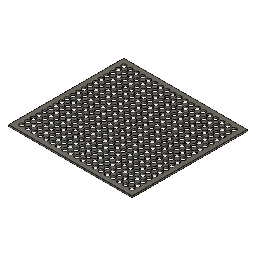
Top (Autodesk Fusion 360 design; units mm, degrees)
Autodesk Fusion 360 part; units mm, degrees
sketch "Sketch1" plane through (0, 0, 0) normal (0, 0, 1) x (1, 0, 0)
  circle A0 centre (11.85, 11) radius 9
  circle A1 centre (35.55, 11) radius 9
  circle A2 centre (59.25, 11) radius 9
  circle A3 centre (82.95, 11) radius 9
  circle A4 centre (106.65, 11) radius 9
  circle A5 centre (130.35, 11) radius 9
  circle A6 centre (154.05, 11) radius 9
  circle A7 centre (177.75, 11) radius 9
  circle A8 centre (201.45, 11) radius 9
  circle A9 centre (225.15, 11) radius 9
  circle A10 centre (248.85, 11) radius 9
  circle A11 centre (272.55, 11) radius 9
  circle A12 centre (296.25, 11) radius 9
  circle A13 centre (319.95, 11) radius 9
  circle A14 centre (343.65, 11) radius 9
  circle A15 centre (367.35, 11) radius 9
  circle A16 centre (391.05, 11) radius 9
  circle A17 centre (414.75, 11) radius 9
  circle A18 centre (438.45, 11) radius 9
  circle A19 centre (11.85, 33) radius 9
  circle A20 centre (35.55, 33) radius 9
  circle A21 centre (59.25, 33) radius 9
  circle A22 centre (82.95, 33) radius 9
  circle A23 centre (106.65, 33) radius 9
  circle A24 centre (130.35, 33) radius 9
  circle A25 centre (154.05, 33) radius 9
  circle A26 centre (177.75, 33) radius 9
  circle A27 centre (201.45, 33) radius 9
  circle A28 centre (225.15, 33) radius 9
  circle A29 centre (248.85, 33) radius 9
  circle A30 centre (272.55, 33) radius 9
  circle A31 centre (296.25, 33) radius 9
  circle A32 centre (319.95, 33) radius 9
  circle A33 centre (343.65, 33) radius 9
  circle A34 centre (367.35, 33) radius 9
  circle A35 centre (391.05, 33) radius 9
  circle A36 centre (414.75, 33) radius 9
  circle A37 centre (438.45, 33) radius 9
  circle A38 centre (11.85, 55) radius 9
  circle A39 centre (35.55, 55) radius 9
  circle A40 centre (59.25, 55) radius 9
  circle A41 centre (82.95, 55) radius 9
  circle A42 centre (106.65, 55) radius 9
  circle A43 centre (130.35, 55) radius 9
  circle A44 centre (154.05, 55) radius 9
  circle A45 centre (177.75, 55) radius 9
  circle A46 centre (201.45, 55) radius 9
  circle A47 centre (225.15, 55) radius 9
  circle A48 centre (248.85, 55) radius 9
  circle A49 centre (272.55, 55) radius 9
  circle A50 centre (296.25, 55) radius 9
  circle A51 centre (319.95, 55) radius 9
  circle A52 centre (343.65, 55) radius 9
  circle A53 centre (367.35, 55) radius 9
  circle A54 centre (391.05, 55) radius 9
  circle A55 centre (414.75, 55) radius 9
  circle A56 centre (438.45, 55) radius 9
  circle A57 centre (11.85, 77) radius 9
  circle A58 centre (35.55, 77) radius 9
  circle A59 centre (59.25, 77) radius 9
  circle A60 centre (82.95, 77) radius 9
  circle A61 centre (106.65, 77) radius 9
  circle A62 centre (130.35, 77) radius 9
  circle A63 centre (154.05, 77) radius 9
  circle A64 centre (177.75, 77) radius 9
  circle A65 centre (201.45, 77) radius 9
  circle A66 centre (225.15, 77) radius 9
  circle A67 centre (248.85, 77) radius 9
  circle A68 centre (272.55, 77) radius 9
  circle A69 centre (296.25, 77) radius 9
  circle A70 centre (319.95, 77) radius 9
  circle A71 centre (343.65, 77) radius 9
  circle A72 centre (367.35, 77) radius 9
  circle A73 centre (391.05, 77) radius 9
  circle A74 centre (414.75, 77) radius 9
  circle A75 centre (438.45, 77) radius 9
  circle A76 centre (11.85, 99) radius 9
  circle A77 centre (35.55, 99) radius 9
  circle A78 centre (59.25, 99) radius 9
  circle A79 centre (82.95, 99) radius 9
  circle A80 centre (106.65, 99) radius 9
  circle A81 centre (130.35, 99) radius 9
  circle A82 centre (154.05, 99) radius 9
  circle A83 centre (177.75, 99) radius 9
  circle A84 centre (201.45, 99) radius 9
  circle A85 centre (225.15, 99) radius 9
  circle A86 centre (248.85, 99) radius 9
  circle A87 centre (272.55, 99) radius 9
  circle A88 centre (296.25, 99) radius 9
  circle A89 centre (319.95, 99) radius 9
  circle A90 centre (343.65, 99) radius 9
  circle A91 centre (367.35, 99) radius 9
  circle A92 centre (391.05, 99) radius 9
  circle A93 centre (414.75, 99) radius 9
  circle A94 centre (438.45, 99) radius 9
  circle A95 centre (11.85, 121) radius 9
  circle A96 centre (35.55, 121) radius 9
  circle A97 centre (59.25, 121) radius 9
  circle A98 centre (82.95, 121) radius 9
  circle A99 centre (106.65, 121) radius 9
  circle A100 centre (130.35, 121) radius 9
  circle A101 centre (154.05, 121) radius 9
  circle A102 centre (177.75, 121) radius 9
  circle A103 centre (201.45, 121) radius 9
  circle A104 centre (225.15, 121) radius 9
  circle A105 centre (248.85, 121) radius 9
  circle A106 centre (272.55, 121) radius 9
  circle A107 centre (296.25, 121) radius 9
  circle A108 centre (319.95, 121) radius 9
  circle A109 centre (343.65, 121) radius 9
  circle A110 centre (367.35, 121) radius 9
  circle A111 centre (391.05, 121) radius 9
  circle A112 centre (414.75, 121) radius 9
  circle A113 centre (438.45, 121) radius 9
  circle A114 centre (11.85, 143) radius 9
  circle A115 centre (35.55, 143) radius 9
  circle A116 centre (59.25, 143) radius 9
  circle A117 centre (82.95, 143) radius 9
  circle A118 centre (106.65, 143) radius 9
  circle A119 centre (130.35, 143) radius 9
  circle A120 centre (154.05, 143) radius 9
  circle A121 centre (177.75, 143) radius 9
  circle A122 centre (201.45, 143) radius 9
  circle A123 centre (225.15, 143) radius 9
  circle A124 centre (248.85, 143) radius 9
  circle A125 centre (272.55, 143) radius 9
  circle A126 centre (296.25, 143) radius 9
  circle A127 centre (319.95, 143) radius 9
  circle A128 centre (343.65, 143) radius 9
  circle A129 centre (367.35, 143) radius 9
  circle A130 centre (391.05, 143) radius 9
  circle A131 centre (414.75, 143) radius 9
  circle A132 centre (438.45, 143) radius 9
  circle A133 centre (11.85, 165) radius 9
  circle A134 centre (35.55, 165) radius 9
  circle A135 centre (59.25, 165) radius 9
  circle A136 centre (82.95, 165) radius 9
  circle A137 centre (106.65, 165) radius 9
  circle A138 centre (130.35, 165) radius 9
  circle A139 centre (154.05, 165) radius 9
  circle A140 centre (177.75, 165) radius 9
  circle A141 centre (201.45, 165) radius 9
  circle A142 centre (225.15, 165) radius 9
  circle A143 centre (248.85, 165) radius 9
  circle A144 centre (272.55, 165) radius 9
  circle A145 centre (296.25, 165) radius 9
  circle A146 centre (319.95, 165) radius 9
  circle A147 centre (343.65, 165) radius 9
  circle A148 centre (367.35, 165) radius 9
  circle A149 centre (391.05, 165) radius 9
  circle A150 centre (414.75, 165) radius 9
  circle A151 centre (438.45, 165) radius 9
  circle A152 centre (11.85, 187) radius 9
  circle A153 centre (35.55, 187) radius 9
  circle A154 centre (59.25, 187) radius 9
  circle A155 centre (82.95, 187) radius 9
  circle A156 centre (106.65, 187) radius 9
  circle A157 centre (130.35, 187) radius 9
  circle A158 centre (154.05, 187) radius 9
  circle A159 centre (177.75, 187) radius 9
  circle A160 centre (201.45, 187) radius 9
  circle A161 centre (225.15, 187) radius 9
  circle A162 centre (248.85, 187) radius 9
  circle A163 centre (272.55, 187) radius 9
  circle A164 centre (296.25, 187) radius 9
  circle A165 centre (319.95, 187) radius 9
  circle A166 centre (343.65, 187) radius 9
  circle A167 centre (367.35, 187) radius 9
  circle A168 centre (391.05, 187) radius 9
  circle A169 centre (414.75, 187) radius 9
  circle A170 centre (438.45, 187) radius 9
  circle A171 centre (11.85, 209) radius 9
  circle A172 centre (35.55, 209) radius 9
  circle A173 centre (59.25, 209) radius 9
  circle A174 centre (82.95, 209) radius 9
  circle A175 centre (106.65, 209) radius 9
  circle A176 centre (130.35, 209) radius 9
  circle A177 centre (154.05, 209) radius 9
  circle A178 centre (177.75, 209) radius 9
  circle A179 centre (201.45, 209) radius 9
  circle A180 centre (225.15, 209) radius 9
  circle A181 centre (248.85, 209) radius 9
  circle A182 centre (272.55, 209) radius 9
  circle A183 centre (296.25, 209) radius 9
  circle A184 centre (319.95, 209) radius 9
  circle A185 centre (343.65, 209) radius 9
  circle A186 centre (367.35, 209) radius 9
  circle A187 centre (391.05, 209) radius 9
  circle A188 centre (414.75, 209) radius 9
  circle A189 centre (438.45, 209) radius 9
  circle A190 centre (11.85, 231) radius 9
  circle A191 centre (35.55, 231) radius 9
  circle A192 centre (59.25, 231) radius 9
  circle A193 centre (82.95, 231) radius 9
  circle A194 centre (106.65, 231) radius 9
  circle A195 centre (130.35, 231) radius 9
  circle A196 centre (154.05, 231) radius 9
  circle A197 centre (177.75, 231) radius 9
  circle A198 centre (201.45, 231) radius 9
  circle A199 centre (225.15, 231) radius 9
  circle A200 centre (248.85, 231) radius 9
  circle A201 centre (272.55, 231) radius 9
  circle A202 centre (296.25, 231) radius 9
  circle A203 centre (319.95, 231) radius 9
  circle A204 centre (343.65, 231) radius 9
  circle A205 centre (367.35, 231) radius 9
  circle A206 centre (391.05, 231) radius 9
  circle A207 centre (414.75, 231) radius 9
  circle A208 centre (438.45, 231) radius 9
  circle A209 centre (11.85, 253) radius 9
  circle A210 centre (35.55, 253) radius 9
  circle A211 centre (59.25, 253) radius 9
  circle A212 centre (82.95, 253) radius 9
  circle A213 centre (106.65, 253) radius 9
  circle A214 centre (130.35, 253) radius 9
  circle A215 centre (154.05, 253) radius 9
  circle A216 centre (177.75, 253) radius 9
  circle A217 centre (201.45, 253) radius 9
  circle A218 centre (225.15, 253) radius 9
  circle A219 centre (248.85, 253) radius 9
  circle A220 centre (272.55, 253) radius 9
  circle A221 centre (296.25, 253) radius 9
  circle A222 centre (319.95, 253) radius 9
  circle A223 centre (343.65, 253) radius 9
  circle A224 centre (367.35, 253) radius 9
  circle A225 centre (391.05, 253) radius 9
  circle A226 centre (414.75, 253) radius 9
  circle A227 centre (438.45, 253) radius 9
  circle A228 centre (11.85, 275) radius 9
  circle A229 centre (35.55, 275) radius 9
  circle A230 centre (59.25, 275) radius 9
  circle A231 centre (82.95, 275) radius 9
  circle A232 centre (106.65, 275) radius 9
  circle A233 centre (130.35, 275) radius 9
  circle A234 centre (154.05, 275) radius 9
  circle A235 centre (177.75, 275) radius 9
  circle A236 centre (201.45, 275) radius 9
  circle A237 centre (225.15, 275) radius 9
  circle A238 centre (248.85, 275) radius 9
  circle A239 centre (272.55, 275) radius 9
  circle A240 centre (296.25, 275) radius 9
  circle A241 centre (319.95, 275) radius 9
  circle A242 centre (343.65, 275) radius 9
  circle A243 centre (367.35, 275) radius 9
  circle A244 centre (391.05, 275) radius 9
  circle A245 centre (414.75, 275) radius 9
  circle A246 centre (438.45, 275) radius 9
  circle A247 centre (11.85, 297) radius 9
  circle A248 centre (35.55, 297) radius 9
  circle A249 centre (59.25, 297) radius 9
  circle A250 centre (82.95, 297) radius 9
  circle A251 centre (106.65, 297) radius 9
  circle A252 centre (130.35, 297) radius 9
  circle A253 centre (154.05, 297) radius 9
  circle A254 centre (177.75, 297) radius 9
  circle A255 centre (201.45, 297) radius 9
  circle A256 centre (225.15, 297) radius 9
  circle A257 centre (248.85, 297) radius 9
  circle A258 centre (272.55, 297) radius 9
  circle A259 centre (296.25, 297) radius 9
  circle A260 centre (319.95, 297) radius 9
  circle A261 centre (343.65, 297) radius 9
  circle A262 centre (367.35, 297) radius 9
  circle A263 centre (391.05, 297) radius 9
  circle A264 centre (414.75, 297) radius 9
  circle A265 centre (438.45, 297) radius 9
  circle A266 centre (11.85, 319) radius 9
  circle A267 centre (35.55, 319) radius 9
  circle A268 centre (59.25, 319) radius 9
  circle A269 centre (82.95, 319) radius 9
  circle A270 centre (106.65, 319) radius 9
  circle A271 centre (130.35, 319) radius 9
  circle A272 centre (154.05, 319) radius 9
  circle A273 centre (177.75, 319) radius 9
  circle A274 centre (201.45, 319) radius 9
  circle A275 centre (225.15, 319) radius 9
  circle A276 centre (248.85, 319) radius 9
  circle A277 centre (272.55, 319) radius 9
  circle A278 centre (296.25, 319) radius 9
  circle A279 centre (319.95, 319) radius 9
  circle A280 centre (343.65, 319) radius 9
  circle A281 centre (367.35, 319) radius 9
  circle A282 centre (391.05, 319) radius 9
  circle A283 centre (414.75, 319) radius 9
  circle A284 centre (438.45, 319) radius 9
  circle A285 centre (11.85, 341) radius 9
  circle A286 centre (35.55, 341) radius 9
  circle A287 centre (59.25, 341) radius 9
  circle A288 centre (82.95, 341) radius 9
  circle A289 centre (106.65, 341) radius 9
  circle A290 centre (130.35, 341) radius 9
  circle A291 centre (154.05, 341) radius 9
  circle A292 centre (177.75, 341) radius 9
  circle A293 centre (201.45, 341) radius 9
  circle A294 centre (225.15, 341) radius 9
  circle A295 centre (248.85, 341) radius 9
  circle A296 centre (272.55, 341) radius 9
  circle A297 centre (296.25, 341) radius 9
  circle A298 centre (319.95, 341) radius 9
  circle A299 centre (343.65, 341) radius 9
  circle A300 centre (367.35, 341) radius 9
  circle A301 centre (391.05, 341) radius 9
  circle A302 centre (414.75, 341) radius 9
  circle A303 centre (438.45, 341) radius 9
  circle A304 centre (11.85, 363) radius 9
  circle A305 centre (35.55, 363) radius 9
  circle A306 centre (59.25, 363) radius 9
  circle A307 centre (82.95, 363) radius 9
  circle A308 centre (106.65, 363) radius 9
  circle A309 centre (130.35, 363) radius 9
  circle A310 centre (154.05, 363) radius 9
  circle A311 centre (177.75, 363) radius 9
  circle A312 centre (201.45, 363) radius 9
  circle A313 centre (225.15, 363) radius 9
  circle A314 centre (248.85, 363) radius 9
  circle A315 centre (272.55, 363) radius 9
  circle A316 centre (296.25, 363) radius 9
  circle A317 centre (319.95, 363) radius 9
  circle A318 centre (343.65, 363) radius 9
  circle A319 centre (367.35, 363) radius 9
  circle A320 centre (391.05, 363) radius 9
  circle A321 centre (414.75, 363) radius 9
  circle A322 centre (438.45, 363) radius 9
  circle A323 centre (11.85, 385) radius 9
  circle A324 centre (35.55, 385) radius 9
  circle A325 centre (59.25, 385) radius 9
  circle A326 centre (82.95, 385) radius 9
  circle A327 centre (106.65, 385) radius 9
  circle A328 centre (130.35, 385) radius 9
  circle A329 centre (154.05, 385) radius 9
  circle A330 centre (177.75, 385) radius 9
  circle A331 centre (201.45, 385) radius 9
  circle A332 centre (225.15, 385) radius 9
  circle A333 centre (248.85, 385) radius 9
  circle A334 centre (272.55, 385) radius 9
  circle A335 centre (296.25, 385) radius 9
  circle A336 centre (319.95, 385) radius 9
  circle A337 centre (343.65, 385) radius 9
  circle A338 centre (367.35, 385) radius 9
  circle A339 centre (391.05, 385) radius 9
  circle A340 centre (414.75, 385) radius 9
  circle A341 centre (438.45, 385) radius 9
  circle A342 centre (11.85, 407) radius 9
  circle A343 centre (35.55, 407) radius 9
  circle A344 centre (59.25, 407) radius 9
  circle A345 centre (82.95, 407) radius 9
  circle A346 centre (106.65, 407) radius 9
  circle A347 centre (130.35, 407) radius 9
  circle A348 centre (154.05, 407) radius 9
  circle A349 centre (177.75, 407) radius 9
  circle A350 centre (201.45, 407) radius 9
  circle A351 centre (225.15, 407) radius 9
  circle A352 centre (248.85, 407) radius 9
  circle A353 centre (272.55, 407) radius 9
  circle A354 centre (296.25, 407) radius 9
  circle A355 centre (319.95, 407) radius 9
  circle A356 centre (343.65, 407) radius 9
  circle A357 centre (367.35, 407) radius 9
  circle A358 centre (391.05, 407) radius 9
  circle A359 centre (414.75, 407) radius 9
  circle A360 centre (438.45, 407) radius 9
  line L0 (0, 0) -> (450.3, 0)
  line L1 (450.3, 0) -> (450.3, 418)
  line L2 (450.3, 418) -> (0, 418)
  line L3 (0, 418) -> (0, 0)
  line L4 (-15, -15) -> (465.3, -15)
  line L5 (465.3, -15) -> (465.3, 433)
  line L6 (465.3, 433) -> (-15, 433)
  line L7 (-15, 433) -> (-15, -15)
  dimension "d3" = 18
  dimension "d8" = 23.7
  dimension "d9" = 22
  dimension "d32" = 450.3
  dimension "d33" = 418
  dimension "d34" = 11.85
  dimension "d35" = 11
  dimension "d36" = 480.3
  dimension "d37" = 448
  dimension "d38" = 15
  dimension "d39" = 15
  constraint horizontal L0
  constraint vertical L1
  constraint horizontal L2
  constraint vertical L3
  constraint coincident L0.start L3.end
  constraint horizontal L4
  constraint vertical L5
  constraint horizontal L6
  constraint vertical L7
  measures "d3" diameter of A0
  measures "d32" distance of L0.start L0.end
  measures "d33" distance of L0.start L2.end
  measures "d34" distance of A0.centre L3
  measures "d35" distance of A0.centre L0
  measures "d36" distance of L4.start L4.end
  measures "d37" distance of L4.start L6.end
  measures "d38" distance of L3 L7
  measures "d39" distance of L0 L4
extrude "Extrude7" add sketch "Sketch1" along normal blind 6.5 contours L0 L1 L2 L3 | L4 L5 L6 L7
named bodies: "Body"
